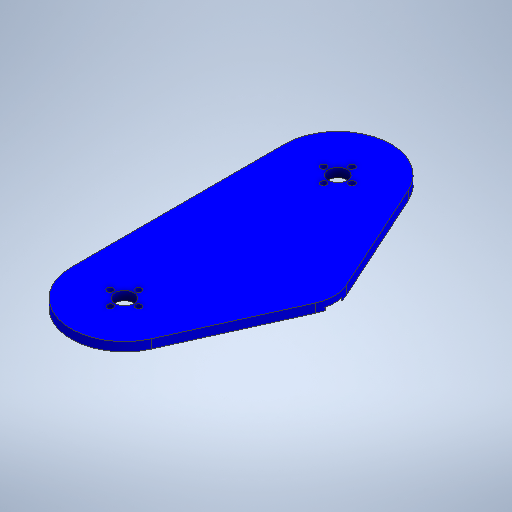
# Autodesk Inventor part: SyringePushMount
Saved by Autodesk Inventor 2025.2 (Build 292293000, 293)
## iProperties
Created: 2025-05-30
Part Number: SyringePushMount
Material: Generic
Document SubType Name: Modeling
Designer: Simon
Density: 1 g/cm^3
Appearance: Default
Author: Simon
Autodesk Inventor part; units mm, degrees
ref_plane "YZ Plane" through (0, 0, 0) normal (1, 0, 0) x (0, 1, 0)
ref_plane "XZ Plane" through (0, 0, 0) normal (0, 1, 0) x (-1, 0, 0)
ref_plane "XY Plane" through (0, 0, 0) normal (0, 0, 1) x (1, 0, 0)
sketch "Sketch1" plane through (0, 0, 0) normal (0, 1, 0) x (-1, 0, 0)
  line L0 (0, 60) -> (0, -60)
  line L1 (0, 0) -> (-60, 0)
  line L2 (-60, 60) -> (-60, -60)
  line L3 (0, 60) -> (-30, 60)
  line L4 (-30, 60) -> (-30, -60)
  arc A0 (0, 60) -> (-60, 60) centre (-30, 60) ccw
  arc A1 (-60, -60) -> (0, -60) centre (-30, -60) ccw
  circle A2 centre (-78, 0) radius 10.5
  line L5 (-30, 60) -> (-38, 60)
  circle A3 centre (-38, 60) radius 1.75
  circle A4 centre (-30, 52) radius 1.75
  circle A5 centre (-22, 60) radius 1.75
  circle A6 centre (-30, 68) radius 1.75
  line L6 (-30, -60) -> (-38, -60)
  circle A7 centre (-38, -60) radius 1.75
  circle A8 centre (-30, -52) radius 1.75
  circle A9 centre (-22, -60) radius 1.75
  circle A10 centre (-30, -68) radius 1.75
  line L7 (-60, 0) -> (-90, 0)
  line L8 (-90, 0) -> (-57.3431, 72.3431)
  line L9 (-90, 0) -> (-57.3431, -72.3431)
  arc A11 (-86.1472, 8.5348) -> (-86.1472, -8.5348) centre (-67.2404, 0) ccw
  line L10 (-90, 0) -> (-78, 0)
  line L11 (-78, 10.5) -> (-85.2601, 10.5)
  line L12 (-78, -10.5) -> (-85.2601, -10.5)
  point P0 (-87.4935, -4.4859)
  point P1 (-87.4935, 4.4859)
  dimension "d0" = 120
  dimension "d1" = 60
  dimension "d2" = 120
  dimension "d5" = 21
  dimension "d15" = 8
  dimension "d16" = 3.5
  dimension "d19" = 360
  dimension "d28" = 30
  dimension "d29" = 12
  constraints: 26 end point, 12 centre point, 10 point on circle, 6 point on line, 6 symmetric about line, 6 tangent, 4 coincident, 3 horizontal, 2 midpoint, 2 vertical, 1 parallel, 1 perpendicular, 13 other
  measures "d0" distance of L0.start L0.end
  measures "d1" distance of L1.start L1.end
  measures "d2" distance of L2.start L2.end
  measures "d5" diameter of A2
  measures "d15" distance of L5.start L5.end
  measures "d16" diameter of A3
  measures "d28" distance of L1.end L7.end
  measures "d29" distance of L7.end L10.end
extrude "Extrusion1" add sketch "Sketch1" along normal blind 5 contours L0 L1 L4 A4 L3 A5 | A3 | L3 A5 L4 A4 L1 L2 A0 | A7 | A8 L4 | L4 A8 | L0 A1 L2 L1 | A5 L3 | L3 A5 | A0 L2 L7 A2 L11 L8 | L11 A2 A11 L8 | L9 L12 A2 L7 L2 A1 | A4 L4 | L4 A4 | A2 L7 A11 | L9 A11 A2 L12 | A2 A11 L7 | A6 | A9 | A10 picked at (-84.0044, 3.1674) picked at (-84.0044, -3.1674)
hole "Hole1" at (30, 0, 60) at (30, 0, -60) direction (0, 1, 0) diameter 10.6 end through all
extrude "Extrusion2" cut sketch "Sketch1" along normal blind 1.5 contours A2 L7 A11 | A2 A11 L7 picked at (-84.0044, 3.1674) picked at (-84.0044, -3.1674)
hole "Hole2" at (38, 0, 60) at (30, 0, 68) at (22, 0, 60) at (30, 0, 52) at (38, 0, -60) at (30, 0, -52) at (30, 0, -68) at (22, 0, -60) direction (0, 1, 0) diameter 3.5 end through all
body "Solid1"
